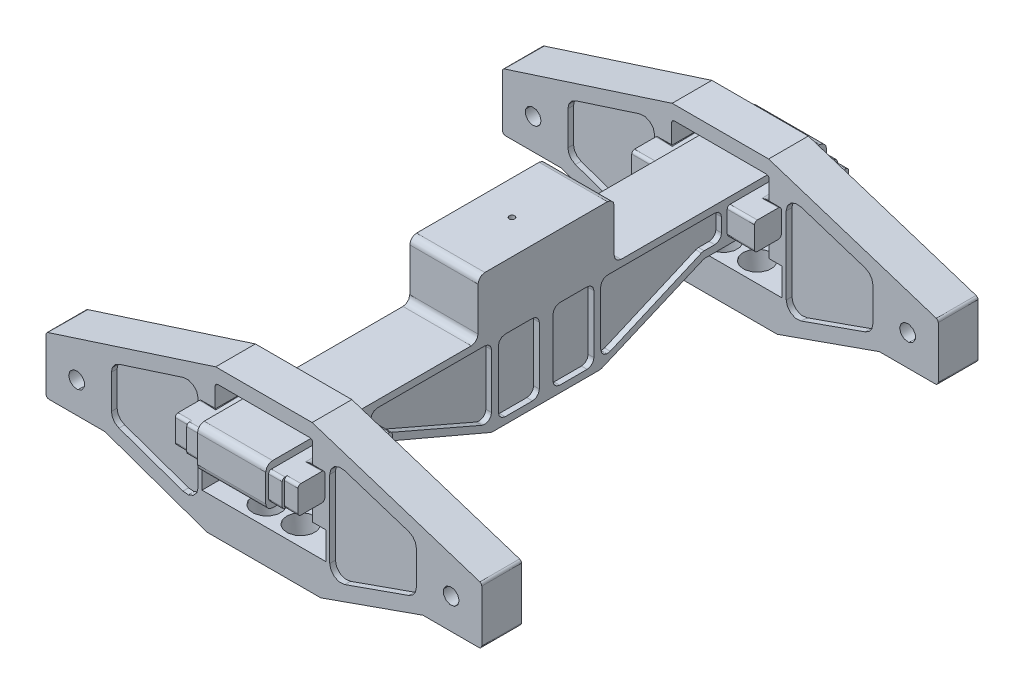
# Autodesk Inventor part: Car_truck
Saved by Autodesk Inventor 2023 (Build 270158000, 158)
## iProperties
Created: 2022-08-16
Part Number: Car_truck
Material: Generic
Document SubType Name: Modeling
Designer: guill
Density: 1 g/cm^3
Appearance: Default
Mass: 662862 g
Surface Area: 184039 cm^2
Volume: 662862 cm^3
Author: guill
## iProperties of the stored document Car_truck_3DPrint.ipt
Created: 2022-10-19
Part Number: Car_truck_3DPrint
Material: Generic
Document SubType Name: Modeling
Designer: guill
Density: 1 g/cm^3
Appearance: Default
Author: guill
Autodesk Inventor part; units mm, degrees
ref_plane "YZ Plane" through (0, 0, 0) normal (1, 0, 0) x (0, 1, 0)
ref_plane "XZ Plane" through (0, 0, 0) normal (0, 1, 0) x (-1, 0, 0)
ref_plane "XY Plane" through (0, 0, 0) normal (0, 0, 1) x (1, 0, 0)
sketch "Sketch1" plane through (0, 0, 0) normal (1, 0, 0) x (0, 1, 0)
  line L0 (635, 0) -> (635, -304.8)
  line L1 (635, -304.8) -> (381, -304.8)
  line L2 (381, -304.8) -> (381, -1255.1874)
  line L3 (381, -1255.1874) -> (197.6438, -1255.1874)
  line L4 (197.6438, -1255.1874) -> (197.6438, -707.2071)
  line L5 (197.6438, -707.2071) -> (0, -244.475)
  line L6 (0, -244.475) -> (0, 0)
  line L7 (0, 0) -> (635, 0)
  dimension "d0" = 304.8
  dimension "d1" = 635
  dimension "d2" = 244.475
  dimension "d3" = 547.9803
  dimension "d4" = 950.3874
  dimension "d5" = 0
  dimension "d6" = 254
  dimension "d7" = 183.3562
  constraints: 16 end point, 2 parallel, 2 perpendicular, 1 horizontal, 1 vertical
  measures "d0" distance of L0.start L0.end
  measures "d1" distance of L6.end L0.start
  measures "d2" distance of L5.end L6.end
  measures "d3" distance of L3.end L4.end
  measures "d4" vertical distance of L3.end L1.end
  measures "d5" vertical distance of L3.end L2.end
  measures "d6" distance of L1.end L0.end
  measures "d7" distance of L3.end L2.end
extrude "Extrusion1" add sketch "Sketch1" along normal mid plane 305.5938
sketch "Sketch2" plane through (152.7969, 0, 0) normal (1, 0, 0) x (0, 0, -1)
  line L0 (60.96, 350.52) -> (183.3562, 350.52)
  line L1 (213.8362, 320.04) -> (213.8362, 60.96)
  line L2 (183.3562, 30.48) -> (60.96, 30.48)
  line L3 (30.48, 60.96) -> (30.48, 320.04)
  line L4 (0, 635) -> (0, 0) projected
  line L5 (0, 0) -> (244.475, 0) projected
  line L6 (1255.1874, 381) -> (304.8, 381) projected
  line L7 (244.3162, 76.8875) -> (244.3162, 320.04)
  line L8 (274.7962, 350.52) -> (754.8074, 350.52)
  line L9 (785.2874, 320.04) -> (785.2874, 258.6038)
  line L10 (1255.1874, 381) -> (1255.1874, 197.6438) projected
  line L11 (754.8074, 228.1238) -> (707.2071, 228.1238)
  line L12 (695.0987, 225.6155) -> (286.9047, 48.9158)
  line L13 (707.2071, 197.6438) -> (1255.1874, 197.6438) projected
  arc A0 (60.96, 350.52) -> (30.48, 320.04) centre (60.96, 320.04) ccw
  arc A1 (213.8362, 320.04) -> (183.3562, 350.52) centre (183.3562, 320.04) ccw
  arc A2 (183.3562, 30.48) -> (213.8362, 60.96) centre (183.3562, 60.96) ccw
  arc A3 (30.48, 60.96) -> (60.96, 30.48) centre (60.96, 60.96) ccw
  arc A4 (244.3162, 76.8875) -> (286.9047, 48.9158) centre (274.7962, 76.8875) ccw
  arc A5 (707.2071, 228.1238) -> (695.0987, 225.6155) centre (707.2071, 197.6438) ccw
  arc A6 (274.7962, 350.52) -> (244.3162, 320.04) centre (274.7962, 320.04) ccw
  arc A7 (754.8074, 228.1238) -> (785.2874, 258.6038) centre (754.8074, 258.6038) ccw
  arc A8 (785.2874, 320.04) -> (754.8074, 350.52) centre (754.8074, 320.04) ccw
  point P0 (30.48, 350.52)
  point P1 (213.8362, 350.52)
  point P2 (30.48, 30.48)
  point P3 (122.2375, 0)
  point P4 (122.1581, 30.48)
  point P5 (244.3162, 30.48)
  point P6 (244.3162, 350.52)
  point P7 (785.2874, 350.52)
  point P8 (785.2874, 228.1238)
  point P9 (700.8931, 228.1238)
  dimension "d13" = 30.48
  dimension "d14" = 30.48
  dimension "d15" = 30.48
  dimension "d16" = 183.3562
  dimension "d17" = 30.48
  dimension "d18" = 30.48
  dimension "d20" = 30.48
  dimension "d24" = 30.48
  dimension "d26" = 30.48
  dimension "d27" = 30.48
  dimension "d43" = 469.9
  dimension "d44" = 469.9
  dimension "d60" = 30.48
  constraints: 18 end point, 18 point on circle, 18 tangent, 16 point on line, 9 centre point, 7 equal radius, 3 parallel, 2 midpoint, 2 perpendicular, 1 horizontal, 1 vertical
  measures "d13" distance from line of L4 point (30.48, 30.48)
  measures "d14" vertical distance of point (122.238, 0) point (122.158, 30.48)
  measures "d15" distance between parallel lines of L6 L0
  measures "d16" distance of point (30.48, 350.52) point (213.836, 350.52)
  measures "d17" distance of point (244.316, 350.52) point (213.836, 350.52)
  measures "d18" distance from line of L6 point (785.287, 350.52)
  measures "d20" distance from line of L13 point (785.287, 228.124)
  measures "d24" vertical distance of L5.end point (244.316, 30.48)
  measures "d26" radius of A0
  measures "d27" radius of A1
  measures "d43" horizontal distance of L10.end point (785.287, 228.124)
  measures "d44" horizontal distance of L10.end point (785.287, 350.52)
  measures "d60" distance from line of L12 L13.start
extrude "Extrusion2" cut sketch "Sketch2" against normal blind 25.4
mirror "Mirror1" about plane through (0, 0, 0) normal (1, 0, 0) of "Extrusion2"
fillet "Fillet1" radius 30.48 6 edges at (0, 635, -304.8) (0, 381, -304.8) (0, 381, -1255.1874) (0, 197.6438, -1255.1874) (0, 197.6438, -707.2071) (0, 0, -244.475)
sketch "Sketch4" plane through (152.7969, 0, 0) normal (1, 0, 0) x (0, 0, -1)
  line L0 (823.3874, 350.52) -> (1229.7874, 350.52)
  line L1 (1242.4874, 337.82) -> (1242.4874, 240.8238)
  line L2 (1255.1874, 228.1238) -> (1255.1874, 350.52) projected
  line L3 (1229.7874, 228.1238) -> (823.3874, 228.1238)
  line L4 (810.6874, 240.8238) -> (810.6874, 337.82)
  line L5 (785.2874, 320.04) -> (785.2874, 258.6038) projected
  line L6 (713.4439, 197.6438) -> (1224.7074, 197.6438) projected
  line L7 (1224.7074, 381) -> (335.28, 381) projected
  arc A0 (823.3874, 350.52) -> (810.6874, 337.82) centre (823.3874, 337.82) ccw
  arc A1 (1242.4874, 337.82) -> (1229.7874, 350.52) centre (1229.7874, 337.82) ccw
  arc A2 (1229.7874, 228.1238) -> (1242.4874, 240.8238) centre (1229.7874, 240.8238) ccw
  arc A3 (810.6874, 240.8238) -> (823.3874, 228.1238) centre (823.3874, 240.8238) ccw
  point P0 (0, 0)
  point P1 (1242.4874, 350.52)
  point P2 (1242.4874, 228.1238)
  point P3 (785.2874, 289.3219)
  dimension "d46" = 25.4
  dimension "d47" = 30.48
  dimension "d48" = 30.48
  dimension "d49" = 12.7
  dimension "d59" = 12.7
  constraints: 8 end point, 8 point on circle, 8 tangent, 4 centre point, 4 point on line, 3 equal radius, 2 parallel, 1 horizontal, 1 midpoint, 1 perpendicular
  measures "d46" distance from line of L4 point (785.287, 289.322)
  measures "d47" distance from line of L6 point (1242.487, 228.124)
  measures "d48" distance from line of L7 point (1242.487, 350.52)
  measures "d49" radius of A0
  measures "d59" distance from line of L2 L1.end
extrude "Extrusion3" add sketch "Sketch4" along normal blind 60.96
mirror "Mirror2" about plane through (0, 0, 0) normal (1, 0, 0) of "Extrusion3"
sketch "Sketch5" plane through (213.7569, 0, 0) normal (1, 0, 0) x (0, 0, -1)
  line L0 (1229.7874, 350.52) -> (823.3874, 350.52) projected
  line L1 (823.3874, 228.1238) -> (1229.7874, 228.1238) projected
  line L2 (823.3874, 350.52) -> (918.1474, 350.52)
  line L3 (930.8474, 337.82) -> (930.8474, 240.8238)
  line L4 (918.1474, 228.1238) -> (823.3874, 228.1238)
  line L5 (810.6874, 240.8238) -> (810.6874, 337.82)
  line L6 (1125.1574, 350.52) -> (1219.9174, 350.52)
  line L7 (1232.6174, 337.82) -> (1232.6174, 240.8238)
  line L8 (1219.9174, 228.1238) -> (1125.1574, 228.1238)
  line L9 (1112.4574, 240.8238) -> (1112.4574, 337.82)
  arc A0 (930.8474, 337.82) -> (918.1474, 350.52) centre (918.1474, 337.82) ccw
  arc A1 (918.1474, 228.1238) -> (930.8474, 240.8238) centre (918.1474, 240.8238) ccw
  arc A2 (1125.1574, 350.52) -> (1112.4574, 337.82) centre (1125.1574, 337.82) ccw
  arc A3 (1112.4574, 240.8238) -> (1125.1574, 228.1238) centre (1125.1574, 240.8238) ccw
  arc A4 (1232.6174, 337.82) -> (1219.9174, 350.52) centre (1219.9174, 337.82) ccw
  arc A5 (1219.9174, 228.1238) -> (1232.6174, 240.8238) centre (1219.9174, 240.8238) ccw
  arc A6 (810.6874, 240.8238) -> (823.3874, 228.1238) centre (823.3874, 240.8238) ccw
  arc A7 (823.3874, 350.52) -> (810.6874, 337.82) centre (823.3874, 337.82) ccw
  line L10 (810.6874, 337.82) -> (810.6874, 240.8238) projected
  point P0 (0, 0)
  point P1 (810.6874, 350.52)
  point P2 (930.8474, 228.1238)
  point P3 (930.8474, 350.52)
  point P4 (810.6874, 228.1238)
  point P5 (1112.4574, 350.52)
  point P6 (1232.6174, 228.1238)
  point P7 (1112.4574, 228.1238)
  point P8 (918.1474, 350.52)
  point P9 (823.3874, 228.1238)
  point P10 (918.1474, 228.1238)
  point P11 (1219.9174, 350.52)
  point P12 (1125.1574, 228.1238)
  point P13 (1219.9174, 228.1238)
  point P14 (1219.9174, 350.52)
  point P15 (1219.9174, 228.1238)
  dimension "d53" = 181.61
  dimension "d54" = 120.16
  dimension "d55" = 120.16
  dimension "d56" = 12.7
  dimension "d57" = 12.7
  dimension "d187" = 0
  constraints: 18 point on line, 16 end point, 16 point on circle, 16 tangent, 8 centre point, 6 equal radius, 4 parallel, 2 horizontal, 2 perpendicular
  measures "d53" distance of point (1112.457, 350.52) point (930.847, 350.52)
  measures "d54" distance of point (930.847, 228.124) point (810.687, 228.124)
  measures "d55" distance of point (1232.617, 228.124) point (1112.457, 228.124)
  measures "d56" radius of A0
  measures "d57" radius of A4
  measures "d187" distance between parallel lines of L10 L5
extrude "Extrusion4" add sketch "Sketch5" along normal blind 60.96 contours A4 L7 A5 L1 A3 L9 A2 L0 | A0 L3 A1 L1 A6 L5 A7 L0
mirror "Mirror3" about plane through (0, 0, 0) normal (1, 0, 0) of "Extrusion4"
fillet "Fillet2" radius 12.7 4 edges at (213.7569, 350.52, -1021.6524) (213.7569, 228.1238, -1021.6524) (-213.7569, 350.52, -1021.6524) (-213.7569, 228.1238, -1021.6524)
sketch "Sketch6" plane through (201.0569, 350.52, -1021.6524) normal (0, 0, 1) x (-1, 0, 0)
  line L0 (201.0569, -152.4) -> (416.9569, -152.4)
  line L1 (416.9569, -152.4) -> (1167.6176, 89.8701)
  line L2 (1176.4169, 101.9562) -> (1176.4169, 334.01)
  line L3 (1163.7169, 346.71) -> (914.7969, 346.71)
  line L4 (910.5718, 347.4334) -> (457.473, 507.2766)
  line L5 (453.2479, 508) -> (201.0569, 508)
  line L6 (353.8537, -30.48) -> (48.26, -30.48) projected
  line L7 (201.0569, 508) -> (201.0569, 356.0762)
  line L8 (201.0569, 356.0762) -> (406.7969, 356.0762)
  line L9 (419.4969, 343.3762) -> (419.4969, -76.2)
  line L10 (406.7969, -88.9) -> (201.0569, -88.9)
  line L11 (201.0569, -88.9) -> (201.0569, -152.4)
  line L12 (353.8537, 122.3962) -> (414.8138, 122.3962) projected
  arc A0 (406.7969, -88.9) -> (419.4969, -76.2) centre (406.7969, -76.2) ccw
  arc A1 (419.4969, 343.3762) -> (406.7969, 356.0762) centre (406.7969, 343.3762) ccw
  arc A2 (457.473, 507.2766) -> (453.2479, 508) centre (453.2479, 495.3) ccw
  arc A3 (910.5718, 347.4334) -> (914.7969, 346.71) centre (914.7969, 359.41) ccw
  arc A4 (1176.4169, 334.01) -> (1163.7169, 346.71) centre (1163.7169, 334.01) ccw
  arc A5 (1167.6176, 89.8701) -> (1176.4169, 101.9562) centre (1163.7169, 101.9562) ccw
  point P0 (0, 0)
  point P1 (1176.4169, 92.71)
  point P2 (1176.4169, 346.71)
  point P3 (912.6224, 346.71)
  point P4 (455.4224, 508)
  point P5 (1039.2569, 346.71)
  point P6 (201.0569, -30.48)
  point P7 (419.4969, 356.0762)
  point P8 (201.0569, -30.48)
  point P9 (402.1137, 134.4045)
  dimension "d74" = 838.2
  dimension "d75" = 215.9
  dimension "d77" = 254
  dimension "d78" = 457.2
  dimension "d80" = 137.16
  dimension "d81" = 161.29
  dimension "d82" = 660.4
  dimension "d85" = 63.5
  dimension "d86" = 218.44
  dimension "d87" = 152.4
  dimension "d88" = 233.68
  dimension "d89" = 12.7
  dimension "d90" = 12.7
  dimension "d130" = 0
  constraints: 22 end point, 12 point on circle, 12 tangent, 11 point on line, 6 centre point, 5 perpendicular, 4 equal radius, 3 midpoint, 2 vertical, 1 horizontal, 1 parallel, 1 other
  measures "d74" horizontal distance of point (1039.257, 346.71) L0.start
  measures "d75" distance of L0.end L0.start
  measures "d77" distance of point (1176.417, 346.71) point (1176.417, 92.71)
  measures "d78" horizontal distance of point (455.422, 508) point (912.622, 346.71)
  measures "d80" distance of point (1176.417, 346.71) point (1039.257, 346.71)
  measures "d81" vertical distance of point (455.422, 508) point (912.622, 346.71)
  measures "d82" distance of L5.end L0.start
  measures "d85" distance of L10.end L0.start
  measures "d86" distance of L7.end point (419.497, 356.076)
  measures "d87" vertical distance of point (0, 0) L0.start
  measures "d89" radius of A0
  measures "d90" radius of A2
  measures "d130" horizontal distance of point (201.057, -30.48) L10.end
extrude "Extrusion6" add sketch "Sketch6" along normal mid plane 177.8 separate body
sketch "Sketch7" plane through (201.0569, 350.52, -1110.5524) normal (0, 0, -1) x (-1, 0, 0)
  line L0 (495.6969, -9.5135) -> (495.6969, -354.667)
  line L1 (563.3972, -402.5734) -> (849.7987, -301.5373)
  line L2 (910.5718, -347.4334) -> (457.473, -507.2766) projected
  line L3 (562.0997, 38.831) -> (848.5013, -53.603)
  line L4 (883.6984, -101.9475) -> (883.6984, -253.6309)
  line L5 (419.4969, 76.2) -> (419.4969, -343.3762) projected
  line L6 (1167.6176, -89.8701) -> (416.9569, 152.4)
  line L7 (1167.6176, -89.8701) -> (416.9569, 152.4) projected
  line L8 (457.473, -507.2766) -> (910.5718, -347.4334) projected
  arc A0 (562.0997, 38.831) -> (495.6969, -9.5135) centre (546.4969, -9.5135) ccw
  arc A1 (883.6984, -101.9475) -> (848.5013, -53.603) centre (832.8984, -101.9475) ccw
  arc A2 (849.7987, -301.5373) -> (883.6984, -253.6309) centre (832.8984, -253.6309) ccw
  arc A3 (495.6969, -354.667) -> (563.3972, -402.5734) centre (546.4969, -354.667) ccw
  point P0 (201.0569, -350.52)
  point P1 (495.6969, 60.262)
  point P2 (495.6969, -426.4565)
  point P3 (883.6984, -289.5782)
  point P4 (883.6984, -64.9626)
  point P5 (684.0224, -427.355)
  point P6 (705.3005, -7.386)
  point P7 (495.6969, 60.262)
  point P8 (883.6984, -64.9626)
  dimension "d93" = 76.2
  dimension "d94" = 63.5
  dimension "d139" = 63.5
  dimension "d140" = 50.8
  constraints: 16 point on line, 10 end point, 8 point on circle, 8 tangent, 4 centre point, 3 equal radius, 2 midpoint, 2 parallel, 2 vertical
  measures "d93" distance from line of L5 point (495.697, -426.457)
  measures "d94" distance from line of point (684.022, -427.355) L1
  measures "d139" distance from line of L6 point (705.3, -7.386)
  measures "d140" radius of A0
extrude "Extrusion7" cut sketch "Sketch7" against normal blind 25.4 bodies 2
mirror "Mirror4" about plane through (201.0569, 350.52, -1021.6524) normal (0, 0, 1) of "Extrusion7" bodies 2
sketch "Sketch8" plane through (201.0569, 350.52, -1110.5524) normal (0, 0, -1) x (-1, 0, 0)
  circle A0 centre (1039.2569, -209.3678) radius 35.6875
  arc A1 (453.2479, -508) -> (457.473, -507.2766) centre (453.2479, -495.3) ccw projected
  line L0 (201.0569, 152.4) -> (201.0569, 88.9) projected
  point P0 (201.0569, -350.52)
  point P1 (455.3912, -507.8178)
  dimension "d103" = 71.375
  dimension "d104" = 298.45
  dimension "d105" = 838.2
  constraints: 1 centre point, 1 point on circle
  measures "d103" diameter of A0
  measures "d104" vertical distance of point (455.391, -507.818) A0.centre
  measures "d105" distance from line of L0 A0.centre
extrude "Extrusion8" cut sketch "Sketch8" against normal through all bodies 2
mirror "Mirror5" about plane through (0, -157.48, -1021.6524) normal (1, 0, 0) bodies 2
mirror "Mirror6" about plane through (0, 635, 0) normal (0, 0, 1) bodies 1 2
sketch "Sketch9" plane through (-152.7969, 635, -274.32) normal (0, 1, 0) x (1, 0, 0)
  circle A0 centre (152.7969, -274.32) radius 12.7
  point P0 (152.7969, -274.32)
  dimension "d108" = 25.4
  constraints: 1 centre point, 1 coincident
  measures "d108" diameter of A0
extrude "Extrusion9" cut sketch "Sketch9" against normal blind 127 bodies 1
sketch "Sketch11" plane through (-205.74, -5.5562, -932.7524) normal (0, 1, 0) x (1, 0, 0)
  circle A0 centre (281.94, 88.9) radius 63.3844
  line L0 (421.64, 177.8) -> (421.64, 0) projected
  line L1 (-10.16, 177.8) -> (421.64, 177.8) projected
  circle A1 centre (129.54, 88.9) radius 63.3844
  point P0 (205.74, -932.7524)
  point P1 (421.64, 88.9)
  point P2 (205.74, 177.8)
  point P3 (205.74, 177.8)
  dimension "d114" = 126.7689
  dimension "d115" = 0
  dimension "d116" = 76.2
  dimension "d117" = 126.7689
  dimension "d118" = 76.2
  dimension "d169" = 0
  constraints: 3 midpoint, 2 centre point
  measures "d114" diameter of A0
  measures "d115" vertical distance of point (421.64, 88.9) A0.centre
  measures "d116" horizontal distance of point (205.74, 177.8) A0.centre
  measures "d117" diameter of A1
  measures "d118" horizontal distance of point (205.74, 177.8) A1.centre
  measures "d169" vertical distance of A0.centre A1.centre
extrude "Extrusion11" cut sketch "Sketch11" along normal blind 352.552 and the other way blind 117.856 bodies 2 1
mirror "Mirror7" about plane through (0, 0, 0) normal (0, 0, 1) of "Extrusion11" bodies 2 1
sketch "Sketch12" plane through (201.0569, 350.52, -1110.5524) normal (0, 0, -1) x (-1, 0, 0)
  line L0 (406.7969, -356.0763) -> (-4.6831, -356.0763) projected
  line L1 (-4.6831, -356.0763) -> (-75.8031, -356.0763)
  line L2 (-75.8031, -356.0763) -> (-75.8031, -232.8863)
  line L3 (-75.8031, -232.8863) -> (-17.3831, -232.8863)
  line L4 (-17.3831, 76.2) -> (-17.3831, -343.3763) projected
  line L5 (48.26, -122.3962) -> (-12.7, -122.3962) projected
  line L6 (48.26, 0) -> (-12.7, 0) projected
  arc A0 (-17.3831, -343.3763) -> (-4.6831, -356.0763) centre (-4.6831, -343.3763) ccw projected
  arc A1 (-17.3831, -343.3763) -> (-4.6831, -356.0763) centre (-4.6831, -343.3762) ccw
  line L7 (-17.3831, -232.8863) -> (-17.3831, -343.3763)
  point P0 (201.0569, -350.52)
  point P1 (-12.7, -122.3962)
  point P2 (-12.7, 0)
  point P3 (17.78, -122.3962)
  point P4 (17.78, 0)
  point P5 (0, -134.4045)
  point P6 (0, -10.7672)
  dimension "d127" = 123.19
  dimension "d131" = 58.42
  constraints: 8 end point, 2 perpendicular, 2 point on circle, 2 tangent, 1 centre point, 1 concentric, 1 horizontal, 1 point on line, 1 vertical, 4 other
  measures "d127" distance of L2.end L1.end
  measures "d131" distance of L3.end L2.end
extrude "Extrusion12" cut sketch "Sketch12" against normal up to surface (177.8 mm away) bodies 2
mirror "Mirror8" about plane through (0, 0, 0) normal (1, 0, 0) of "Extrusion12" bodies 2
mirror "Mirror9" about plane through (0, 0, 0) normal (0, 0, 1) of "Extrusion12", "Mirror8" bodies 2
scale "Scale1" factors (0.042277, 0.042277, 0.042277) then translate (-72.9785, 260.8069, 978.46) bodies 1 2
body "Solid1"
body "Solid3"
